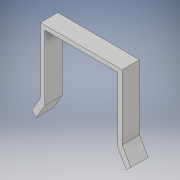
# Autodesk Inventor part: U-Part Gen 2
Saved by Autodesk Inventor 2019 (Build 230136000, 136)
## iProperties
Created: 2019-10-05
Part Number: U-Part Gen 2
Material: Generic
Document SubType Name: Modeling
Designer: Delta
Density: 1 g/cm^3
Appearance: Default
Author: Delta
Autodesk Inventor part; units mm, degrees
ref_plane "YZ Plane" through (0, 0, 0) normal (1, 0, 0) x (0, 1, 0)
ref_plane "XZ Plane" through (0, 0, 0) normal (0, 1, 0) x (-1, 0, 0)
ref_plane "XY Plane" through (0, 0, 0) normal (0, 0, 1) x (1, 0, 0)
sketch "Sketch1" plane through (0, 0, 0) normal (0, 0, 1) x (1, 0, 0)
  line L0 (0, 0) -> (119.38, 0)
  line L1 (119.38, 0) -> (119.38, -6.35)
  line L2 (119.38, -6.35) -> (0, -6.35)
  line L3 (0, -6.35) -> (0, 0)
  line L4 (119.38, 0) -> (113.03, 0)
  line L5 (113.03, 0) -> (113.03, -101.6)
  line L6 (113.03, -101.6) -> (119.38, -101.6)
  line L7 (119.38, -101.6) -> (119.38, 0)
  line L8 (0, 0) -> (6.35, 0)
  line L9 (6.35, 0) -> (6.35, -101.6)
  line L10 (6.35, -101.6) -> (0, -101.6)
  line L11 (0, -101.6) -> (0, 0)
  line L12 (0, -95.25) -> (-12.7, -117.247)
  line L13 (0, -95.25) -> (25.4, -95.25) construction
  line L14 (6.35, -101.6) -> (-6.35, -123.597)
  line L15 (6.35, -101.6) -> (31.75, -101.6) construction
  line L16 (-6.35, -123.597) -> (-12.7, -117.247)
  dimension "d0" = 119.38
  dimension "d1" = 6.35
  dimension "d2" = 6.35
  dimension "d3" = 101.6
  dimension "d4" = 6.35
  dimension "d5" = 101.6
  dimension "d6" = 6.35
  dimension "d7" = 120
  dimension "d8" = 12.7
  dimension "d9" = 25.4
  dimension "d10" = 120
  constraints: 34 end point, 6 parallel, 5 horizontal, 3 perpendicular, 2 equal length, 1 point on line
  measures "d0" distance of L1.end L2.end
  measures "d1" distance of L0.end L1.end
  measures "d2" distance of L6.end L5.end
  measures "d3" distance of L5.end L4.end
  measures "d4" distance between parallel lines of L9 L11
  measures "d5" distance between parallel lines of L10 L0
  measures "d6" distance of L12.start L10.end
  measures "d7" angle of L12 L13
  measures "d8" horizontal distance of L12.start L12.end
  measures "d9" distance of L9.end L14.end
  measures "d10" angle of L14 L15
extrude "Extrusion1" add sketch "Sketch1" along normal blind 25.4
ref_plane "Work Plane1" through (59.69, -101.6, 0) normal (1, 0, 0) x (0, 0, -1)
mirror "Mirror1" about plane through (59.69, -101.6, 0) normal (1, 0, 0) of "Extrusion1"
equation "\"d2\" = d1"
equation "\"d4\" = d1"
equation "\"d5\" = d3"
equation "\"d6\" = d4"
body "Solid1"
